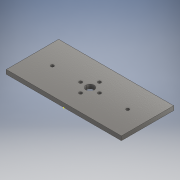
# Autodesk Inventor part: frontal
Saved by Autodesk Inventor 2018 (Build 220112000, 112)
## iProperties
Created: 2019-04-02
Part Number: frontal
Material: Acero, galvanizado
Document SubType Name: Modeling
Designer: Victor Hernandez
Density: 7.85 g/cm^3
Appearance: Galvanizado
Author: Victor Hernandez
Autodesk Inventor part; units mm, degrees
ref_plane "YZ Plane" through (0, 0, 0) normal (1, 0, 0) x (0, 1, 0)
ref_plane "XZ Plane" through (0, 0, 0) normal (0, 1, 0) x (-1, 0, 0)
ref_plane "XY Plane" through (0, 0, 0) normal (0, 0, 1) x (1, 0, 0)
sketch "Boceto1" plane through (0, 0, 0) normal (0, 0, 1) x (1, 0, 0)
  line L0 (-27.5, -12.5) -> (27.5, -12.5)
  line L1 (27.5, -12.5) -> (27.5, 12.5)
  line L2 (27.5, 12.5) -> (-27.5, 12.5)
  line L3 (-27.5, 12.5) -> (-27.5, -12.5)
  line L4 (-27.5, -12.5) -> (27.5, 12.5) construction
  line L5 (27.5, -12.5) -> (-27.5, 12.5) construction
  circle A0 centre (0, 0) radius 2
  circle A1 centre (0, -4.5) radius 0.75
  circle A2 centre (0, 4.5) radius 0.75
  circle A3 centre (4.5, 0) radius 0.75
  circle A4 centre (-4.5, 0) radius 0.75
  line L6 (0, 0) -> (18, 0) construction
  line L7 (0, 0) -> (18, 0) construction
  circle A5 centre (-18, 0) radius 0.75
  circle A6 centre (18, 0) radius 0.75
  dimension "d0" = 55
  dimension "d1" = 25
  dimension "d2" = 4
  dimension "d4" = 1.5
  dimension "d8" = 1.5
  dimension "d9" = 1.5
  dimension "d10" = 1.5
  dimension "d15" = 1.5
  dimension "d16" = 1.5
  constraints: 16 end point, 7 centre point, 3 horizontal, 2 coincident, 2 midpoint, 2 parallel, 1 perpendicular
  measures "d0" distance of L2.end L1.end
  measures "d1" distance of L1.end L0.end
  measures "d2" diameter of A0
  measures "d4" diameter of A1
  measures "d8" diameter of A2
  measures "d9" diameter of A3
  measures "d10" diameter of A4
  measures "d15" diameter of A5
  measures "d16" diameter of A6
extrude "Extrusión1" add sketch "Boceto1" along normal blind 2
sketch "Boceto2" plane through (0, 0, 0) normal (1, 0, 0) x (0, 1, 0)
  point P0 (-12.5, 0)
